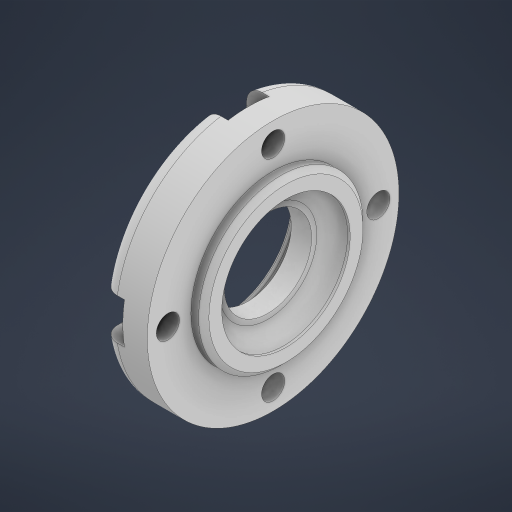
# Autodesk Inventor part: 부품3
Saved by Autodesk Inventor 2023 (Build 270158000, 158)
## iProperties
Created: 2022-11-14
Part Number: 부품3
Material: 일반
Document SubType Name: Modeling
Designer: LJH
Density: 1 g/cm^3
Appearance: 기본값
Author: LJH
Autodesk Inventor part; units mm, degrees
ref_plane "YZ Plane" through (0, 0, 0) normal (1, 0, 0) x (0, 1, 0)
ref_plane "XZ Plane" through (0, 0, 0) normal (0, 1, 0) x (-1, 0, 0)
ref_plane "XY Plane" through (0, 0, 0) normal (0, 0, 1) x (1, 0, 0)
sketch "스케치1" plane through (0, 0, 0) normal (0, 0, 1) x (1, 0, 0)
  line L0 (-5.8319, 24.5) -> (5.8319, 24.5)
  line L1 (5.8319, 24.5) -> (5.8319, 8.5)
  line L2 (5.8319, 8.5) -> (-5.8319, 8.5)
  line L3 (-5.8319, 8.5) -> (-5.8319, 24.5)
  line L4 (-5.8319, 24.5) -> (5.8319, 8.5) construction
  line L5 (5.8319, 24.5) -> (-5.8319, 8.5) construction
  line L6 (5.8319, 8.5) -> (2.3319, 8.5)
  line L7 (2.3319, 8.5) -> (2.3319, 12.5)
  line L8 (2.3319, 12.5) -> (5.8319, 12.5)
  line L9 (5.8319, 12.5) -> (5.8319, 8.5)
  line L10 (-5.8319, 8.5) -> (-1.6319, 8.5)
  line L11 (-1.6319, 8.5) -> (-1.6319, 12.5)
  line L12 (-1.6319, 12.5) -> (-5.8319, 12.5)
  line L13 (-5.8319, 12.5) -> (-5.8319, 8.5)
  line L14 (5.8319, 24.5) -> (3.3319, 24.5)
  line L15 (3.3319, 24.5) -> (3.3319, 16)
  line L16 (3.3319, 16) -> (5.8319, 16)
  line L17 (5.8319, 16) -> (5.8319, 24.5)
  line L18 (-8.1647, 0) -> (8.1647, 0) projected
  point P0 (0, 0)
  point P1 (0, 16.5)
  dimension "d0" = 8.5
  dimension "d1" = 16
  dimension "d2" = 3.5
  dimension "d3" = 4
  dimension "d4" = 4.2
  dimension "d5" = 4
  dimension "d6" = 2.5
  dimension "d7" = 8.5
  constraints: 36 end point, 8 parallel, 4 horizontal, 4 perpendicular, 2 midpoint
  measures "d0" distance from line of point (0, 0) L2
  measures "d1" distance of L0.end L1.end
  measures "d2" distance of L7.end L8.end
  measures "d3" distance of L6.end L7.end
  measures "d4" distance of L12.end L11.end
  measures "d5" distance of L11.end L10.end
  measures "d6" distance of L16.end L15.end
  measures "d7" distance of L15.end L14.end
revolve "회전1" add sketch "스케치1" angle 360 about axis through (-10, 0, 0) along (1, 0, 0) contours L0 L15 L16 L1 L8 L7 L2 L11 L12 L3
sketch "스케치2" plane through (-5.8319, 0, 0) normal (-1, 0, 0) x (0, 0, 1)
  circle A0 centre (0, 0) radius 20.5
  circle A1 centre (0, 20.5) radius 4
  circle A2 centre (0, 20.5) radius 2.25
  line L0 (4, 20.5) -> (-4, 20.5)
  line L1 (-4, 20.5) -> (-4, 27.4124)
  line L2 (-4, 27.4124) -> (4, 27.4124)
  line L3 (4, 27.4124) -> (4, 20.5)
  dimension "d9" = 41
  dimension "d10" = 8
  dimension "d11" = 4.5
  constraints: 8 end point, 2 coincident, 2 parallel, 1 centre point, 1 horizontal, 1 perpendicular, 1 vertical alignment, 5 other
  measures "d11" diameter of A2
extrude "돌출1" cut sketch "스케치2" against normal blind 4.4 contours A1 A0 A2 | A0 A2 L0 A1 | A1 L0 A2 A0 | A2 A0 | A0 L0 A2 | L0 A2 A1 | A1 L1 L2 L3 | A2 L0 A0 | L0 A2
extrude "돌출2" cut sketch "스케치2" against normal blind 15.4 contours A2 A0 | A0 L0 A2 | A2 L0 A0 | L0 A2
pattern_circular "원형 패턴1" count 4 over 360 about axis through (-1.25, 0, 0) along (1, 0, 0) of "돌출1", "돌출2"
fillet "모깎기1" radius 3 5 edges at (-5.8319, 17.3241, -17.3241) (-5.8319, -17.3241, -17.3241) (-5.8319, -17.3241, 17.3241) (-5.8319, 17.3241, 17.3241) (2.3319, -12.5, 0)
chamfer "모따기1" distance 1 angle 45 1 edges at (5.8319, -16, 0)
fillet "모깎기2" radius 0.5 1 edges at (-1.6319, -12.5, 0)
chamfer "모따기2" distance 0.6 angle 20 1 edges at (-5.8319, -12.5, 0) measured on face at (-5.3319, -12.5, 0)
fillet "모깎기3" radius 2 1 edges at (-5.2319, -12.5, 0)
